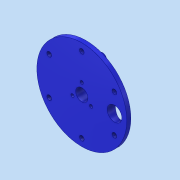
# Autodesk Inventor part: pistonSealingWallRear
Saved by Autodesk Inventor 2017 (Build 210142000, 142)
## iProperties
Created: 2016-11-26
Part Number: pistonSealingWallRear
Material: ABS Plastic
Document SubType Name: Modeling
Designer: techn
Density: 1.06 g/cm^3
Appearance: Blue - Wall Paint - Glossy
Author: techn
Autodesk Inventor part; units mm, degrees
ref_plane "YZ Plane" through (0, 0, 0) normal (1, 0, 0) x (0, 1, 0)
ref_plane "XZ Plane" through (0, 0, 0) normal (0, 1, 0) x (-1, 0, 0)
ref_plane "XY Plane" through (0, 0, 0) normal (0, 0, 1) x (1, 0, 0)
sketch "Sketch1" plane through (0, 0, 0) normal (0, 0, 1) x (1, 0, 0)
  circle A0 centre (0, 0) radius 34.925
  dimension "d0" = 69.85
  constraints: 1 centre point, 1 coincident
  measures "d0" diameter of A0
extrude "Extrusion1" add sketch "Sketch1" along normal blind 3.175
sketch "Sketch4" plane through (0, 0, 0) normal (1, 0, 0) x (0, 1, 0)
  line L0 (-34.925, 0) -> (34.925, 0) projected
  line L1 (34.925, 0) -> (33.02, 0)
  line L2 (0, 0) -> (0, -9.525)
  line L3 (0, -9.525) -> (11.1125, -9.525)
  arc A0 (33.02, 0) -> (11.1125, -9.525) centre (33.02, -29.9561) ccw
  line L4 (0, 0) -> (19.05, 0)
  dimension "d15" = 1.905
  dimension "d16" = 9.525
  dimension "d17" = 11.1125
  dimension "d39" = 19.05
  constraints: 8 end point, 2 point on circle, 2 point on line, 1 centre point, 1 perpendicular, 1 tangent, 1 vertical
  measures "d15" distance of L0.end L1.end
  measures "d16" distance of L2.start L2.end
  measures "d17" distance of L2.end L3.end
  measures "d39" distance of L2.start L4.end
revolve "Revolution1" add sketch "Sketch4" angle 360 about axis through (0, 0, 0) along (0, 0, -1)
sketch "Sketch2" plane through (0, 0, 3.175) normal (0, 0, 1) x (1, 0, 0)
  line L0 (0, 0) -> (0, 29.21)
  circle A0 centre (0, 29.21) radius 1.8415
  circle A1 centre (-25.2966, 14.605) radius 1.8415
  circle A2 centre (-25.2966, -14.605) radius 1.8415
  circle A3 centre (0, -29.21) radius 1.8415
  circle A4 centre (25.2966, -14.605) radius 1.8415
  circle A5 centre (25.2966, 14.605) radius 1.8415
  dimension "d3" = 29.21
  dimension "d4" = 3.683
  dimension "d7" = 360
  constraints: 6 centre point, 2 end point, 1 coincident, 1 vertical, 13 other
  measures "d3" distance of L0.start L0.end
  measures "d4" diameter of A0
extrude "Extrusion2" cut sketch "Sketch2" against normal blind 4.7625
sketch "Sketch5" plane through (0, 0, 0) normal (0, 0, -1) x (-1, 0, 0)
  spline S0 degree 2 poles (-1.8415, 29.21) (-1.8415, 32.3996) (0.9207, 30.8048) (3.683, 29.21) (0.9208, 27.6152) (-1.8415, 26.0204) (-1.8415, 29.21) knots 0 0 0 0.333333 0.333333 0.666667 0.666667 1 1 1 weights 1 0.5 1 0.5 1 0.5 1 projected
  circle A0 centre (0, 29.21) radius 1.8415 projected
  circle A1 centre (0, 29.21) radius 3.175
  circle A2 centre (-25.2966, 14.605) radius 3.175
  circle A3 centre (-25.2966, -14.605) radius 3.175
  circle A4 centre (0, -29.21) radius 3.175
  circle A5 centre (25.2966, -14.605) radius 3.175
  circle A6 centre (25.2966, 14.605) radius 3.175
  spline S1 degree 2 poles (-27.1381, 14.605) (-27.1381, 17.7946) (-24.3759, 16.1998) (-21.6136, 14.605) (-24.3759, 13.0102) (-27.1381, 11.4154) (-27.1381, 14.605) knots 0 0 0 0.333333 0.333333 0.666667 0.666667 1 1 1 weights 1 0.5 1 0.5 1 0.5 1 projected
  spline S2 degree 2 poles (-27.1381, -14.605) (-27.1381, -11.4154) (-24.3759, -13.0102) (-21.6136, -14.605) (-24.3759, -16.1998) (-27.1381, -17.7946) (-27.1381, -14.605) knots 0 0 0 0.333333 0.333333 0.666667 0.666667 1 1 1 weights 1 0.5 1 0.5 1 0.5 1 projected
  spline S3 degree 2 poles (-1.8415, -29.21) (-1.8415, -26.0204) (0.9208, -27.6152) (3.683, -29.21) (0.9208, -30.8048) (-1.8415, -32.3996) (-1.8415, -29.21) knots 0 0 0 0.333333 0.333333 0.666667 0.666667 1 1 1 weights 1 0.5 1 0.5 1 0.5 1 projected
  spline S4 degree 2 poles (23.4551, -14.605) (23.4551, -11.4154) (26.2174, -13.0102) (28.9796, -14.605) (26.2174, -16.1998) (23.4551, -17.7946) (23.4551, -14.605) knots 0 0 0 0.333333 0.333333 0.666667 0.666667 1 1 1 weights 1 0.5 1 0.5 1 0.5 1 projected
  spline S5 degree 2 poles (23.4551, 14.605) (23.4551, 17.7946) (26.2174, 16.1998) (28.9796, 14.605) (26.2174, 13.0102) (23.4551, 11.4154) (23.4551, 14.605) knots 0 0 0 0.333333 0.333333 0.666667 0.666667 1 1 1 weights 1 0.5 1 0.5 1 0.5 1 projected
  point P0 (0, 0)
  dimension "d19" = 6.35
  dimension "d22" = 360
  constraints: 6 centre point, 1 coincident, 1 vertical alignment, 19 other
  measures "d19" diameter of A1
extrude "Extrusion4" add sketch "Sketch5" along normal blind 1.5875
sketch "Sketch6" plane through (0, 0, -9.525) normal (0, 0, -1) x (-1, 0, 0)
  circle A0 centre (0, 0) radius 4.7625
  line L0 (0, 0) -> (0, 8.3295)
  circle A1 centre (0, 8.3295) radius 1.27
  circle A2 centre (-7.2136, -4.1648) radius 1.27
  circle A3 centre (7.2136, -4.1648) radius 1.27
  dimension "d26" = 9.525
  dimension "d27" = 2.54
  dimension "d30" = 360
  dimension "d32" = 14.4272
  constraints: 4 centre point, 2 coincident, 2 end point, 1 vertical, 7 other
  measures "d26" diameter of A0
  measures "d27" diameter of A1
  measures "d32" distance of A3.centre L0.end
extrude "Extrusion5" cut sketch "Sketch6" against normal through all
sketch "Sketch7" plane through (0, 0, 3.175) normal (0, 0, 1) x (1, 0, 0)
  line L0 (0, 0) -> (25.4, 0)
  circle A0 centre (25.4, 0) radius 5.715
  dimension "d35" = 25.4
  dimension "d36" = 11.43
  constraints: 2 end point, 1 centre point, 1 coincident, 1 horizontal
  measures "d35" distance of L0.start L0.end
  measures "d36" diameter of A0
extrude "Extrusion6" cut sketch "Sketch7" against normal through all
sketch "Sketch8" plane through (0, 0, 0) normal (0, 0, -1) x (-1, 0, 0)
  circle A0 centre (0, 0) radius 4.7625 projected
  line L0 (0, 0) -> (-9.7732, 26.8517)
  line L1 (0, 0) -> (28.575, 0) construction
  circle A1 centre (-9.7732, 26.8517) radius 3.175
  point P0 (0, 0)
  dimension "d40" = 28.575
  dimension "d41" = 110
  dimension "d42" = 6.35
  constraints: 4 end point, 1 centre point, 1 coincident, 1 equal length, 1 horizontal
  measures "d40" distance of L0.start L0.end
  measures "d41" angle of L1 L0
  measures "d42" diameter of A1
extrude "Extrusion7" add sketch "Sketch8" along normal blind 3.175 contours A1
fillet "Fillet1" radius 1.27 2 edges at (12.6698, 28.1518, -0.0771) (6.8817, 25.5402, -0.7291)
body "Solid1"
